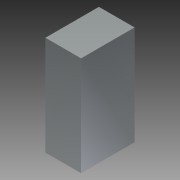
# Autodesk Inventor part: AllowedEnvelope
Saved by Autodesk Inventor 2015 (Build 190159000, 159)
## iProperties
Created: 2015-01-24
Part Number: AllowedEnvelope
Material: Glass
Document SubType Name: Modeling
Designer: pltwe4
Density: 2.18 g/cm^3
Appearance: Clear
Author: pltwe4
Autodesk Inventor part; units mm, degrees
ref_plane "YZ Plane" through (0, 0, 0) normal (1, 0, 0) x (0, 1, 0)
ref_plane "XZ Plane" through (0, 0, 0) normal (0, 1, 0) x (-1, 0, 0)
ref_plane "XY Plane" through (0, 0, 0) normal (0, 0, 1) x (1, 0, 0)
sketch "Sketch1" plane through (0, 0, 0) normal (0, 1, 0) x (-1, 0, 0)
  line L0 (-355.6, 533.4) -> (355.6, 533.4)
  line L1 (355.6, 533.4) -> (355.6, -533.4)
  line L2 (355.6, -533.4) -> (-355.6, -533.4)
  line L3 (-355.6, -533.4) -> (-355.6, 533.4)
  line L4 (-497.84, 0) -> (497.84, 0) projected
  line L5 (0, -746.76) -> (0, 746.76) projected
  point P0 (0, 0)
  dimension "d0" = 711.2
  dimension "d1" = 1066.8
  constraints: 8 end point, 2 parallel, 1 horizontal, 1 perpendicular, 2 other
  measures "d0" distance of L0.start L0.end
  measures "d1" distance of L0.start L2.end
extrude "Extrusion1" add sketch "Sketch1" along normal blind 1981.2
body "Solid1"
